Autodesk Fusion 360 part; units mm, degrees
(part 2 of 2)
sketch "Skizze6 (2)" plane through (0, 6, 0) normal (0, -1, 0) x (1, 0, 0) in component "cutouts"
  line L0 (82, 5) -> (172, 5)
  line L1 (172, 5) -> (172, 50)
  line L2 (172, 50) -> (82, 50)
  line L3 (82, 50) -> (82, 5)
  line L4 (87, 10) -> (167, 10)
  line L5 (167, 10) -> (167, 45)
  line L6 (167, 45) -> (87, 45)
  line L7 (87, 45) -> (87, 10)
  line L8 (92.4157, 47.7212) -> (96.4157, 47.7212)
  line L9 (96.4157, 47.7212) -> (96.4157, 6.7721)
  line L10 (96.4157, 6.7721) -> (92.4157, 6.7721)
  line L11 (92.4157, 6.7721) -> (92.4157, 47.7212)
  line L12 (105.7014, 47.7212) -> (105.7014, 6.7721)
  line L13 (101.7014, 6.7721) -> (101.7014, 47.7212)
  line L14 (114.9871, 47.7212) -> (114.9871, 6.7721)
  line L15 (110.9871, 6.7721) -> (110.9871, 47.7212)
  line L16 (124.2728, 47.7212) -> (124.2728, 6.7721)
  line L17 (120.2728, 6.7721) -> (120.2728, 47.7212)
  line L18 (133.5585, 47.7212) -> (133.5585, 6.7721)
  line L19 (129.5585, 6.7721) -> (129.5585, 47.7212)
  line L20 (142.8443, 47.7212) -> (142.8443, 6.7721)
  line L21 (138.8443, 6.7721) -> (138.8443, 47.7212)
  line L22 (152.13, 47.7212) -> (152.13, 6.7721)
  line L23 (148.13, 6.7721) -> (148.13, 47.7212)
  line L24 (161.4157, 47.7212) -> (161.4157, 6.7721)
  line L25 (157.4157, 6.7721) -> (157.4157, 47.7212)
  line L26 (157.4157, 36) -> (105.7014, 36)
  line L27 (105.7014, 40) -> (157.4157, 40)
  line L28 (0, 10) -> (178, 10)
  dimension "d245" = -5
  dimension "d246" = 4
  dimension "d249" = 65
  dimension "d250" = 0
  dimension "d405" = 4
  dimension "d408" = 3.2279
  dimension "d409" = 5
  constraint horizontal L8
  constraint vertical L9
  constraint horizontal L10
  constraint vertical L11
  constraint coincident L25 L26.start
  constraint perpendicular L16 L26
  constraint coincident L25 L27.end
  constraint perpendicular L25 L27
  constraint coincident L12 L26.end
  measures "d246" distance of L8.start L8.end
  measures "d405" distance of L26.end L27.start
  measures "d408" distance of L10 L28
  measures "d409" distance of L6 L27
extrude "Extrusion8'''" cut sketch "Skizze6 (2)" against normal blind 10 contours L4 L6 L7 L11 L28 | L4 L5 L6 L24 L28 | L4 L6 L9 L13 L28 | L4 L22 L25 L26 L28 | L4 L22 L23 L26 L28 | L6 L22 L25 L27 | L4 L12 L15 L26 L28 | L4 L20 L23 L26 L28 | L12 L15 L26 L27 | L6 L12 L15 L27 | L4 L20 L21 L26 L28 | L6 L20 L23 L27 | L4 L14 L17 L26 L28 | L4 L18 L21 L26 L28 | L4 L16 L17 L26 L28 | L6 L14 L17 L27 | L4 L18 L19 L26 L28 | L6 L18 L21 L27 | L4 L16 L19 L26 L28 | L6 L16 L19 L27 bodies 5 in component "computer-case"
sketch "Skizze7" plane through (82, 0, 0) normal (-1, 0, 0) x (0, -1, 0) in component "cutouts"
  line L0 (-19.5, 8) -> (-19.5, 28)
  line L1 (-19.5, 28) -> (-9, 28)
  line L2 (-9, 28) -> (-9, 8)
  line L3 (-9, 8) -> (-19.5, 8)
  line L4 (-169, 5) -> (-6, 5)
  line L5 (-6, 5) -> (-6, 50)
  line L6 (-6, 50) -> (-169, 50)
  line L7 (-169, 50) -> (-169, 5)
  line L8 (-137.7003, 5) -> (-137.7003, 50)
  line L9 (-166, 13) -> (-146, 13)
  line L10 (-146, 13) -> (-146, 33)
  line L11 (-146, 33) -> (-166, 33)
  line L12 (-166, 33) -> (-166, 13)
  dimension "d253" = 20
  dimension "d254" = 20
  dimension "d255" = 8
  dimension "d256" = 3
  constraint horizontal L9
  constraint vertical L10
  constraint horizontal L11
  constraint vertical L12
  measures "d253" distance of L9.start L9.end
  measures "d254" distance of L9.start L11.end
  measures "d255" distance of L4 L9.start
  measures "d256" distance of L7 L12
extrude "Extrusion10''" cut sketch "Skizze7" along normal blind 14 from surface at -10 contours L9 L10 L11 L12 bodies 7 in component "power-supply"
extrude "Extrusion9''" cut sketch "Skizze7" along normal blind 14 from surface at -10 contours L9 L10 L11 L12 bodies 5 in component "computer-case"
sketch "Skizze8" plane through (0, 137.7003, 0) normal (0, 1, 0) x (-1, 0, 0) in component "cutouts"
  line L0 (-81, 5) -> (-6, 5)
  line L1 (-6, 5) -> (-6, 50)
  line L2 (-6, 50) -> (-81, 50)
  line L3 (-81, 50) -> (-81, 5)
  line L4 (-66, 28) -> (-21, 28)
  line L5 (-21, 28) -> (-21, 8)
  line L6 (-21, 8) -> (-66, 8)
  line L7 (-66, 8) -> (-66, 28)
  line L8 (-21, 28) -> (-6, 28) construction
  line L9 (-66, 28) -> (-81, 28) construction
  circle A0 centre (-77.5, 8.5) radius 1
  circle A1 centre (-9.5, 8.5) radius 1
  circle A2 centre (-77.5, 8.5) radius 2.5
  circle A3 centre (-9.5, 8.5) radius 2.5
  dimension "d287" = 45
  dimension "d288" = 20
  dimension "d289" = 3
  dimension "d296" = 5
  dimension "d297" = 5
  constraint horizontal L4
  constraint vertical L5
  constraint horizontal L6
  constraint vertical L7
  constraint coincident L1 L8.end
  constraint perpendicular L1 L8
  constraint coincident L3 L9.end
  constraint perpendicular L3 L9
  constraint equal L8 L9
  constraint concentric A0 A2
  constraint concentric A1 A3
  measures "d287" distance of L4.start L4.end
  measures "d288" distance of L4.start L6.end
  measures "d289" distance of L0 L6
  measures "d296" diameter of A2
  measures "d297" diameter of A3
extrude "Extrusion15" cut sketch "Skizze8" along normal blind 15 from surface at -8 contours L4 L5 L6 L7 bodies 2 in component "light-controller-case"
extrude "Extrusion11'" cut sketch "Skizze8" along normal blind 15 from surface at -8 contours L4 L5 L6 L7 bodies 8 in component "power-supply"
extrude "Extrusion16" cut sketch "Skizze8" against normal blind 2 contours A0 | A1 | A2 | A3 bodies 2 in component "light-controller-case"
sketch "Skizze4 (4)" plane through (0, 0, 113) normal (0, 0, 1) x (-1, 0, 0) in component "fan-holder"
  line L0 (-13.419, -136.793) -> (-138.419, -136.793)
  line L1 (-138.419, -136.793) -> (-138.419, -162.9077)
  line L2 (-138.419, -162.9077) -> (-82, -162.9077)
  line L3 (-82, -162.9077) -> (-82, -137.7003)
  line L4 (-82, -137.7003) -> (-13.419, -137.7003)
  line L5 (-13.419, -137.7003) -> (-13.419, -136.793)
  ellipse E0 centre (-75.919, -81.793) end of major axis (-132.919, -81.793) minor radius 50.9823
  line L6 (-138.419, -26.793) -> (-138.419, -136.793)
  line L7 (-138.419, -136.793) -> (-13.419, -136.793)
  line L8 (-13.419, -136.793) -> (-13.419, -26.793)
  line L9 (-13.419, -26.793) -> (-138.419, -26.793)
  line L10 (-133.419, -31.793) -> (-133.419, -131.793) construction
  line L11 (-133.419, -131.793) -> (-18.419, -131.793) construction
  line L12 (-18.419, -131.793) -> (-18.419, -31.793) construction
  line L13 (-18.419, -31.793) -> (-133.419, -31.793) construction
  circle A0 centre (-133.419, -131.793) radius 1
  circle A1 centre (-18.419, -131.793) radius 1
  circle A2 centre (-18.419, -31.793) radius 1
  circle A3 centre (-133.419, -31.793) radius 1
  ellipse E1 centre (-127.919, -35.2828) end of major axis (-128.919, -35.2828) minor radius 0.8944
  ellipse E2 centre (-127.919, -128.3032) end of major axis (-128.919, -128.3032) minor radius 0.8944
  ellipse E3 centre (-23.919, -35.2828) end of major axis (-24.919, -35.2828) minor radius 0.8944
  ellipse E4 centre (-23.919, -128.3032) end of major axis (-24.919, -128.3032) minor radius 0.8944
  circle A4 centre (-18.419, -131.793) radius 2.5
  circle A5 centre (-133.419, -131.793) radius 2.5
  circle A6 centre (-133.419, -31.793) radius 2.5
  circle A7 centre (-18.419, -31.793) radius 2.5
  dimension "d300" = -5
  dimension "d301" = 2
  dimension "d302" = 2
  dimension "d303" = 2
  dimension "d304" = 2
  dimension "d315" = 5
  dimension "d316" = 5
  dimension "d317" = 5
  dimension "d318" = 5
  constraint coincident L10.end L11.start
  constraint coincident L11.end L12.start
  constraint coincident L12.end L13.start
  constraint coincident L10.start L13.end
  constraint concentric A1 A4
  constraint concentric A0 A5
  constraint concentric A3 A6
  constraint concentric A2 A7
  measures "d301" diameter of A0
  measures "d302" diameter of A1
  measures "d303" diameter of A2
  measures "d304" diameter of A3
  measures "d315" diameter of A4
  measures "d316" diameter of A5
  measures "d317" diameter of A6
  measures "d318" diameter of A7
extrude "Extrusion4'''" cut sketch "Skizze4 (4)" against normal blind 55 contours A0 | A1 | A2 | A3 | A4 | A5 | A6 | A7 bodies 9 in component "fan-holder"
extrude "Extrusion18" cut sketch "Skizze4 (4)" against normal blind 70 contours A0 | A1 | A2 | A3 bodies 4 in component "light-controller-case"
extrude "Extrusion11''" cut sketch "Skizze4 (4)" against normal blind 70 contours A0 | A1 | A2 | A3 bodies 6 in component "computer-case"
extrude "Extrusion5'''" cut sketch "Skizze4 (4)" against normal blind 70 contours A0 | A1 | A2 | A3 bodies 9 in component "fan-holder"
extrude "Extrusion9'''" cut sketch "Skizze2 (3)" against normal blind 20 contours L26 L27 L28 L29 bodies 1 in component "case"
extrude "Extrusion12'" cut sketch "Skizze2 (3)" against normal blind 20 contours L26 L27 L28 L29 bodies 7 in component "power-supply"
sketch "Skizze9" plane through (0, 138.7003, 0) normal (0, -1, 0) x (1, 0, 0) in component "cutouts"
  line L0 (66, 28) -> (66, 8)
  line L1 (66, 8) -> (21, 8)
  line L2 (21, 8) -> (21, 28)
  line L3 (21, 28) -> (66, 28)
  line L4 (47.5027, 53) -> (47.5027, 93.0501)
  spline S0 degree 3 poles (47.5027, 93.0501) (47.5194, 93.0724) (47.5362, 93.0947) (47.553, 93.117) (49.0347, 95.0847) (50.6133, 96.9794) (52.3027, 98.7588) knots -4.432405 -4.432405 -4.432405 -4.432405 -4.42386 -4.42386 -4.42386 -3.669325 -3.669325 -3.669325 -3.669325
  line L5 (44.5027, 88.7668) -> (44.5027, 53)
  line L6 (44.5027, 53) -> (39.7027, 53)
  line L7 (39.7027, 53) -> (39.7027, 80.5615)
  spline S1 degree 3 poles (39.7027, 80.5615) (40.3231, 81.743) (40.9644, 82.9128) (42.5424, 85.6635) (43.4988, 87.232) (44.5027, 88.7668) knots -5.933426 -5.933426 -5.933426 -5.933426 -5.526632 -5.526632 -4.965959 -4.965959 -4.965959 -4.965959
  line L8 (60.1027, 53) -> (55.3027, 53)
  line L9 (55.3027, 53) -> (55.3027, 101.6818)
  spline S2 degree 3 poles (55.3027, 101.6818) (55.3993, 101.7685) (55.4962, 101.8548) (56.7256, 102.9409) (57.9048, 103.8871) (59.4535, 104.9916) (59.7765, 105.2148) (60.1027, 105.4328) knots -3.239152 -3.239152 -3.239152 -3.239152 -3.199117 -3.199117 -2.733019 -2.733019 -2.611699 -2.611699 -2.611699 -2.611699
  line L10 (36.7027, 74.4264) -> (36.7027, 53)
  line L11 (36.7027, 53) -> (31.9027, 53)
  line L12 (31.9027, 53) -> (31.9027, 62.5142)
  spline S3 degree 3 poles (31.9027, 62.5142) (33.2964, 66.4358) (34.8355, 70.2996) (36.5988, 74.198) (36.6507, 74.3123) (36.7027, 74.4264) knots -7.929108 -7.929108 -7.929108 -7.929108 -6.665095 -6.665095 -6.626914 -6.626914 -6.626914 -6.626914
  line L13 (63.1027, 53) -> (63.1027, 107.2351)
  line L14 (76, 108) -> (76, 53)
  line L15 (67.9027, 53) -> (63.1027, 53)
  circle A0 centre (9.5, 109.5) radius 1
  circle A1 centre (9.5, 8.5) radius 1
  circle A2 centre (77.5, 109.5) radius 1
  circle A3 centre (77.5, 8.5) radius 1
  line L16 (6, 5) -> (81, 5)
  line L17 (81, 5) -> (81, 113)
  line L18 (81, 113) -> (6, 113)
  line L19 (6, 113) -> (6, 5)
  line L20 (6, 53) -> (81, 53)
  line L21 (11, 55) -> (21, 55)
  line L22 (21, 55) -> (21, 62)
  line L23 (21, 62) -> (11, 62)
  line L24 (11, 62) -> (11, 55)
  line L25 (64.6301, 108) -> (67.9027, 108)
  line L26 (52.3027, 98.7588) -> (52.3027, 53)
  line L27 (52.3027, 53) -> (47.5027, 53)
  line L28 (60.1027, 105.4328) -> (60.1027, 53)
  spline S4 degree 3 poles (63.1027, 107.2351) (63.6055, 107.5036) (64.1147, 107.759) (64.6301, 108) knots -2.249901 -2.249901 -2.249901 -2.249901 -2.072733 -2.072733 -2.072733 -2.072733
  line L29 (67.9027, 108) -> (67.9027, 53)
  line L30 (76, 53) -> (70.9027, 53)
  line L31 (70.9027, 53) -> (70.9027, 108)
  line L32 (70.9027, 108) -> (76, 108)
  dimension "d333" = 10
  dimension "d334" = 7
  dimension "d335" = 2
  dimension "d336" = 5
  constraint horizontal L21
  constraint vertical L22
  constraint horizontal L23
  constraint vertical L24
  measures "d333" distance of L21.start L21.end
  measures "d334" distance of L21.start L23.end
  measures "d335" distance of L20 L21
  measures "d336" distance of L19 L24
extrude "Extrusion13'" cut sketch "Skizze9" against normal blind 10 contours L21 L22 L23 L24 bodies 8 in component "power-supply"
sketch "Skizze1 (6)" plane through (0, 0, 53) normal (0, 0, 1) x (-1, 0, 0) in component "arduino-mega-case"
  circle A0 centre (-133.419, -31.793) radius 1
  circle A1 centre (-133.419, -131.793) radius 1
  line L0 (-132.5453, -90.7579) -> (-132.5453, -105.3281)
  ellipse E0 centre (-75.919, -98.043) end of major axis (-75.919, -34.3151) minor radius 57 (-132.5453, -90.7579) -> (-132.5453, -105.3281) ccw
  line L1 (-121.2953, -59.4751) -> (-121.2953, -136.6109)
  ellipse E1 centre (-75.919, -98.043) end of major axis (-75.919, -34.3151) minor radius 57 (-128.5453, -122.5244) -> (-121.2953, -136.6109) ccw
  line L2 (-128.5453, -122.5244) -> (-128.5453, -73.5617)
  ellipse E2 centre (-75.919, -98.043) end of major axis (-75.919, -34.3151) minor radius 57 (-121.2953, -59.4751) -> (-128.5453, -73.5617) ccw
  line L3 (-94.7953, -158.175) -> (-94.7953, -37.911)
  ellipse E3 centre (-75.919, -98.043) end of major axis (-75.919, -34.3151) minor radius 57 (-88.0723, -35.7805) -> (-94.7953, -37.911) ccw
  line L4 (-88.0723, -35.7805) -> (-88.0723, -160.3055)
  ellipse E4 centre (-75.919, -98.043) end of major axis (-75.919, -34.3151) minor radius 57 (-94.7953, -158.175) -> (-88.0723, -160.3055) ccw
  line L5 (-110.0453, -46.999) -> (-110.0453, -149.087)
  ellipse E5 centre (-75.919, -98.043) end of major axis (-75.919, -34.3151) minor radius 57 (-117.2953, -141.8751) -> (-110.0453, -149.087) ccw
  line L6 (-117.2953, -141.8751) -> (-117.2953, -54.211)
  ellipse E6 centre (-75.919, -98.043) end of major axis (-75.919, -34.3151) minor radius 57 (-110.0453, -46.999) -> (-117.2953, -54.211) ccw
  line L7 (-98.7953, -39.6727) -> (-98.7953, -156.4133)
  ellipse E7 centre (-75.919, -98.043) end of major axis (-75.919, -34.3151) minor radius 57 (-106.0453, -152.1425) -> (-98.7953, -156.4133) ccw
  line L8 (-106.0453, -152.1425) -> (-106.0453, -43.9435)
  ellipse E8 centre (-75.919, -98.043) end of major axis (-75.919, -34.3151) minor radius 57 (-98.7953, -39.6727) -> (-106.0453, -43.9435) ccw
  ellipse E9 centre (-127.919, -39.9052) end of major axis (-127.919, -38.7872) minor radius 1 (-127.1786, -39.1537) -> (-128.6593, -39.1537) ccw
  line L9 (-127.1786, -39.1537) -> (-128.6593, -39.1537)
  circle A2 centre (-168.5, -165.5) radius 1
  circle A3 centre (-168.5, -9.5) radius 1
  circle A4 centre (-85.5, -9.5) radius 1
  circle A5 centre (-85.5, -165.5) radius 1
  line L10 (-82, -6) -> (-172, -6)
  line L11 (-172, -6) -> (-172, -169)
  line L12 (-172, -169) -> (-82, -169)
  line L13 (-82, -169) -> (-82, -6)
  line L14 (-138.419, -26.793) -> (-138.419, -136.793)
  line L15 (-171, -161.774) -> (-143.419, -161.774)
  line L16 (-143.419, -161.774) -> (-143.419, -26.774)
  line L17 (-143.419, -26.774) -> (-171, -26.774)
  line L18 (-171, -26.774) -> (-171, -161.774)
  line L19 (-168, -158.774) -> (-146.419, -158.774)
  line L20 (-146.419, -158.774) -> (-146.419, -29.774)
  line L21 (-146.419, -29.774) -> (-168, -29.774)
  line L22 (-168, -29.774) -> (-168, -158.774)
  line L23 (-146.419, -29.774) -> (-146.419, -26.774)
  line L24 (-146.419, -158.774) -> (-146.419, -161.774)
  line L25 (-152.0037, -35.3587) -> (-162.4153, -35.3587) construction
  line L26 (-162.4153, -35.3587) -> (-162.4153, -153.1893) construction
  line L27 (-162.4153, -153.1893) -> (-152.0037, -153.1893) construction
  line L28 (-152.0037, -153.1893) -> (-152.0037, -35.3587) construction
  circle A6 centre (-162.4153, -153.1893) radius 1
  circle A7 centre (-152.0037, -153.1893) radius 1
  circle A8 centre (-162.4153, -35.3587) radius 1
  circle A9 centre (-152.0037, -35.3587) radius 1
  circle A10 centre (-162.4153, -35.3587) radius 2.5
  circle A11 centre (-152.0037, -35.3587) radius 2.5
  circle A12 centre (-162.4153, -153.1893) radius 2.5
  circle A13 centre (-152.0037, -153.1893) radius 2.5
  dimension "d339" = 1
  dimension "d340" = 5
  dimension "d341" = 135
  dimension "d342" = 20.774
  dimension "d343" = -3
  dimension "d362" = -8.5847
  dimension "d363" = 2
  dimension "d364" = 2
  dimension "d365" = 2
  dimension "d366" = 2
  dimension "d367" = 5
  dimension "d368" = 5
  dimension "d369" = 5
  dimension "d370" = 5
  constraint horizontal L15
  constraint vertical L16
  constraint horizontal L17
  constraint vertical L18
  constraint coincident L17 L23.end
  constraint perpendicular L17 L23
  constraint coincident L15 L24.end
  constraint perpendicular L15 L24
  constraint coincident L26.end L27.start
  constraint coincident L27.end L28.start
  constraint coincident L25.end L26.start
  constraint coincident L25.start L28.end
  constraint concentric A8 A10
  constraint concentric A9 A11
  constraint concentric A6 A12
  constraint concentric A7 A13
  measures "d339" distance of L11 L18
  measures "d340" distance of L14 L16
  measures "d341" distance of L15.start L17.end
  measures "d342" distance of L10 L17.end
  measures "d363" diameter of A6
  measures "d364" diameter of A7
  measures "d365" diameter of A8
  measures "d366" diameter of A9
  measures "d367" diameter of A10
  measures "d368" diameter of A11
  measures "d369" diameter of A12
  measures "d370" diameter of A13
extrude "Extrusion1''''" add sketch "Skizze1 (6)" along normal blind 60 separate body contours L15 L17 L18 L19 L21 L22 L23 L24 makes body 10 in component "arduino-mega-case"
extrude "Extrusion2''''" add sketch "Skizze1 (6)" along normal blind 3 contours L19 L20 L21 L22 | A6 | A7 | A8 | A9 | A10 | A11 | A12 | A13 bodies 10 in component "arduino-mega-case"
extrude "Extrusion3''''" add sketch "Skizze1 (6)" along normal blind 3 from surface at 60 contours L15 L17 L18 L19 L21 L22 L23 L24 | L19 L20 L21 L22 | A6 | A7 | A8 | A9 | A10 | A11 | A12 | A13 bodies 10 in component "arduino-mega-case"
extrude "Extrusion4''''" add sketch "Skizze1 (6)" along normal blind 63 separate body contours L15 L16 L17 L20 L23 L24 makes body 11 in component "arduino-mega-case"
chamfer "Fase1'''''" distance 6 angle 45 4 edges at (157.2095, 158.774, 56) (157.2095, 158.774, 113) (157.2095, 29.774, 56) (157.2095, 29.774, 113) on bodies 10 in component "arduino-mega-case"
sketch "Skizze3 (4)" plane through (146.419, 0, 0) normal (-1, 0, 0) x (0, -1, 0) in component "arduino-mega-case"
  line L0 (-29.774, 62) -> (-35.774, 56)
  line L1 (-35.774, 56) -> (-152.774, 56)
  line L2 (-152.774, 56) -> (-158.774, 62)
  line L3 (-158.774, 62) -> (-158.774, 107)
  line L4 (-158.774, 107) -> (-152.774, 113)
  line L5 (-152.774, 113) -> (-35.774, 113)
  line L6 (-35.774, 113) -> (-29.774, 107)
  line L7 (-29.774, 107) -> (-29.774, 62)
  line L8 (-26.774, 53) -> (-26.774, 116)
  line L9 (-26.774, 116) -> (-161.774, 116)
  line L10 (-161.774, 116) -> (-161.774, 53)
  line L11 (-161.774, 53) -> (-26.774, 53)
  line L12 (-158.274, 56.5) -> (-30.274, 56.5) construction
  line L13 (-30.274, 56.5) -> (-30.274, 112.5) construction
  line L14 (-30.274, 112.5) -> (-158.274, 112.5) construction
  line L15 (-158.274, 112.5) -> (-158.274, 56.5) construction
  circle A0 centre (-30.274, 112.5) radius 1
  circle A1 centre (-30.274, 56.5) radius 1
  circle A2 centre (-158.274, 56.5) radius 1
  circle A3 centre (-158.274, 112.5) radius 1
  dimension "d354" = -3.5
  dimension "d355" = 2
  dimension "d356" = 2
  dimension "d357" = 2
  dimension "d358" = 2
  constraint coincident L13.end L14.start
  constraint coincident L12.end L13.start
  constraint coincident L12.start L15.end
  constraint coincident L14.end L15.start
  measures "d355" diameter of A0
  measures "d356" diameter of A1
  measures "d357" diameter of A2
  measures "d358" diameter of A3
extrude "Extrusion5''''" cut sketch "Skizze3 (4)" along normal blind 10 from surface at -7 contours A0 | A1 | A2 | A3 bodies 10 11 in component "arduino-mega-case"
extrude "Extrusion6''''" cut sketch "Skizze1 (6)" along normal blind 15 contours A6 | A7 | A8 | A9 bodies 10 in component "arduino-mega-case"
extrude "Extrusion7''''" cut sketch "Skizze1 (6)" along normal blind 11 from surface at 3 contours A10 | A11 | A12 | A13 bodies 10 in component "arduino-mega-case"
sketch "Skizze10" plane through (0, 26.774, 0) normal (0, -1, 0) x (1, 0, 0) in component "cutouts"
  line L0 (146.419, 53) -> (171, 53)
  line L1 (171, 53) -> (171, 116)
  line L2 (171, 116) -> (146.419, 116)
  line L3 (146.419, 116) -> (146.419, 53)
  line L4 (151.419, 111) -> (151.419, 58)
  line L5 (151.419, 58) -> (166, 58)
  line L6 (166, 58) -> (166, 111)
  line L7 (166, 111) -> (151.419, 111)
  dimension "d376" = -5
extrude "Extrusion8''''" cut sketch "Skizze10" against normal blind 10 contours L4 L5 L6 L7 bodies 10 in component "arduino-mega-case"
sketch "Skizze11" plane through (0, 0, 53) normal (0, 0, 1) x (-1, 0, 0) in component "cutouts"
  circle A0 centre (-133.419, -31.793) radius 1
  circle A1 centre (-133.419, -131.793) radius 1
  line L0 (-132.5453, -90.7579) -> (-132.5453, -105.3281)
  ellipse E0 centre (-75.919, -98.043) end of major axis (-75.919, -34.3151) minor radius 57 (-132.5453, -90.7579) -> (-132.5453, -105.3281) ccw
  line L1 (-121.2953, -59.4751) -> (-121.2953, -136.6109)
  ellipse E1 centre (-75.919, -98.043) end of major axis (-75.919, -34.3151) minor radius 57 (-128.5453, -122.5244) -> (-121.2953, -136.6109) ccw
  line L2 (-128.5453, -122.5244) -> (-128.5453, -73.5617)
  ellipse E2 centre (-75.919, -98.043) end of major axis (-75.919, -34.3151) minor radius 57 (-121.2953, -59.4751) -> (-128.5453, -73.5617) ccw
  line L3 (-94.7953, -158.175) -> (-94.7953, -37.911)
  ellipse E3 centre (-75.919, -98.043) end of major axis (-75.919, -34.3151) minor radius 57 (-88.0723, -35.7805) -> (-94.7953, -37.911) ccw
  line L4 (-88.0723, -35.7805) -> (-88.0723, -160.3055)
  ellipse E4 centre (-75.919, -98.043) end of major axis (-75.919, -34.3151) minor radius 57 (-94.7953, -158.175) -> (-88.0723, -160.3055) ccw
  line L5 (-110.0453, -46.999) -> (-110.0453, -149.087)
  ellipse E5 centre (-75.919, -98.043) end of major axis (-75.919, -34.3151) minor radius 57 (-117.2953, -141.8751) -> (-110.0453, -149.087) ccw
  line L6 (-117.2953, -141.8751) -> (-117.2953, -54.211)
  ellipse E6 centre (-75.919, -98.043) end of major axis (-75.919, -34.3151) minor radius 57 (-110.0453, -46.999) -> (-117.2953, -54.211) ccw
  line L7 (-98.7953, -39.6727) -> (-98.7953, -156.4133)
  ellipse E7 centre (-75.919, -98.043) end of major axis (-75.919, -34.3151) minor radius 57 (-106.0453, -152.1425) -> (-98.7953, -156.4133) ccw
  line L8 (-106.0453, -152.1425) -> (-106.0453, -43.9435)
  ellipse E8 centre (-75.919, -98.043) end of major axis (-75.919, -34.3151) minor radius 57 (-98.7953, -39.6727) -> (-106.0453, -43.9435) ccw
  ellipse E9 centre (-127.919, -39.9052) end of major axis (-127.919, -38.7872) minor radius 1 (-127.1786, -39.1537) -> (-128.6593, -39.1537) ccw
  line L9 (-127.1786, -39.1537) -> (-128.6593, -39.1537)
  circle A2 centre (-168.5, -165.5) radius 1
  circle A3 centre (-168.5, -9.5) radius 1
  circle A4 centre (-85.5, -9.5) radius 1
  circle A5 centre (-85.5, -165.5) radius 1
  line L10 (-82, -6) -> (-172, -6)
  line L11 (-172, -6) -> (-172, -169)
  line L12 (-172, -169) -> (-82, -169)
  line L13 (-82, -169) -> (-82, -6)
  line L14 (-166, -26.774) -> (-151.419, -26.774)
  line L15 (-151.419, -26.774) -> (-151.419, -12.193)
  line L16 (-151.419, -12.193) -> (-166, -12.193)
  line L17 (-166, -12.193) -> (-166, -26.774)
  constraint coincident L14.end L15.start
  constraint perpendicular L14 L15
  constraint perpendicular L15 L16
  constraint coincident L14.start L17.end
  constraint equal L14 L15
extrude "Extrusion12''" cut sketch "Skizze11" against normal blind 10 contours L14 L15 L16 L17 bodies 6 in component "computer-case"
sketch "Skizze4 (5)" plane through (168, 0, 0) normal (-1, 0, 0) x (0, -1, 0) in component "arduino-mega-case"
  line L0 (-29.774, 107) -> (-35.774, 113)
  line L1 (-35.774, 113) -> (-152.774, 113)
  line L2 (-152.774, 113) -> (-158.774, 107)
  line L3 (-158.774, 107) -> (-158.774, 62)
  line L4 (-158.774, 62) -> (-152.774, 56)
  line L5 (-152.774, 56) -> (-35.774, 56)
  line L6 (-35.774, 56) -> (-29.774, 62)
  line L7 (-29.774, 62) -> (-29.774, 107)
  circle A0 centre (-158.274, 112.5) radius 1
  circle A1 centre (-158.274, 56.5) radius 1
  circle A2 centre (-30.274, 112.5) radius 1
  circle A3 centre (-30.274, 56.5) radius 1
  line L8 (-29.774, 62) -> (-35.774, 56)
  line L9 (-35.774, 56) -> (-152.774, 56)
  line L10 (-152.774, 56) -> (-158.774, 62)
  line L11 (-158.774, 62) -> (-158.774, 107)
  line L12 (-158.774, 107) -> (-152.774, 113)
  line L13 (-152.774, 113) -> (-35.774, 113)
  line L14 (-35.774, 113) -> (-29.774, 107)
  line L15 (-29.774, 107) -> (-29.774, 62)
  line L16 (-26.774, 53) -> (-26.774, 116)
  line L17 (-26.774, 116) -> (-161.774, 116)
  line L18 (-161.774, 116) -> (-161.774, 53)
  line L19 (-161.774, 53) -> (-26.774, 53)
  line L20 (-50.6836, 57.87) -> (-151.9836, 57.87) construction
  line L21 (-151.9836, 57.87) -> (-151.9836, 111.13) construction
  line L22 (-151.9836, 111.13) -> (-50.6836, 111.13) construction
  line L23 (-50.6836, 111.13) -> (-50.6836, 57.87) construction
  line L24 (-50.6836, 57.87) -> (-151.9836, 111.13) construction
  line L25 (-151.9836, 57.87) -> (-50.6836, 111.13) construction
  line L26 (-161.774, 84.5) -> (-26.774, 84.5) construction
  line L27 (-151.9836, 60.11) -> (-50.6836, 60.11) construction
  line L28 (-151.9836, 108.75) -> (-50.6836, 108.75) construction
  circle A4 centre (-64.9936, 108.75) radius 1
  circle A5 centre (-65.6836, 60.11) radius 1
  circle A6 centre (-140.7036, 60.11) radius 1
  circle A7 centre (-147.3336, 108.75) radius 1
  point P0 (-101.3336, 84.5)
  dimension "d381" = 101.3
  dimension "d382" = 53.26
  dimension "d383" = 2.24
  dimension "d384" = 2.38
  dimension "d385" = 2
  dimension "d386" = 2
  dimension "d387" = 2
  dimension "d388" = 2
  dimension "d389" = 14.31
  dimension "d390" = 15
  dimension "d391" = 4.65
  dimension "d392" = 11.28
  constraint horizontal L20
  constraint perpendicular L20 L21
  constraint parallel L20 L22
  constraint parallel L21 L23
  constraint coincident L24 P0
  constraint coincident L25 P0
  constraint midpoint L18 L26.start
  constraint midpoint L16 L26.end
  constraint coincident L21 L27.start
  constraint coincident L23 L27.end
  constraint perpendicular L23 L27
  constraint coincident L21 L28.start
  constraint coincident L23 L28.end
  constraint perpendicular L23 L28
  constraint coincident L28 A4.centre
  constraint coincident L27 A5.centre
  constraint coincident L27 A6.centre
  constraint coincident L28 A7.centre
  measures "d381" distance of L21.end L22.end
  measures "d382" distance of L20.end L21.end
  measures "d383" distance of L20 L27
  measures "d384" distance of L22 L28
  measures "d385" diameter of A4
  measures "d386" diameter of A5
  measures "d387" diameter of A6
  measures "d388" diameter of A7
  measures "d389" distance of L28.end A4.centre
  measures "d390" distance of L27.end A5.centre
  measures "d391" distance of L28.start A7.centre
  measures "d392" distance of L27.start A6.centre
extrude "Extrusion9''''" cut sketch "Skizze4 (5)" against normal blind 15 contours A4 | A5 | A6 | A7 bodies 10 in component "arduino-mega-case"
sketch "Skizze5 (3)" plane through (0, 169, 0) normal (0, 1, 0) x (-1, 0, 0) in component "computer-case"
  line L0 (-172, 5) -> (-82, 5)
  line L1 (-82, 5) -> (-82, 50)
  line L2 (-82, 50) -> (-172, 50)
  line L3 (-172, 50) -> (-172, 5)
  line L4 (-162, 36) -> (-92, 36)
  line L5 (-92, 36) -> (-92, 8)
  line L6 (-92, 8) -> (-162, 8)
  line L7 (-162, 8) -> (-162, 36)
  dimension "d395" = 3
  dimension "d396" = 14
  dimension "d397" = 10
  dimension "d398" = 10
  constraint horizontal L4
  constraint vertical L5
  constraint horizontal L6
  constraint vertical L7
  measures "d395" distance of L0 L6
  measures "d396" distance of L2 L4
  measures "d397" distance of L1 L5
  measures "d398" distance of L3 L7
extrude "Extrusion10'''" cut sketch "Skizze5 (3)" along normal blind 20 from surface at -5 contours L4 L5 L6 L7 bodies 1 in component "case"
extrude "Extrusion13''" cut sketch "Skizze5 (3)" along normal blind 20 from surface at -5 contours L4 L5 L6 L7 bodies 5 in component "computer-case"
extrude "Extrusion14'" cut 1 faces at (36, 140.7003, 8) along direction (0, 0, -1) blind 6 on bodies 8 bodies 8 in component "power-supply"
component "case" placed x (1, 0, 0) y (0, 1, 0) z (0, 0, 1) at (0, 0, 0)
component "light-controller-case" placed x (1, 0, 0) y (0, 1, 0) z (0, 0, 1) at (0, 0, 0)
component "computer-case" placed x (1, 0, 0) y (0, 1, 0) z (0, 0, 1) at (0, 0, 0)
component "power-supply" placed x (1, 0, 0) y (0, 1, 0) z (0, 0, 1) at (0, 0, 0)
component "fan-holder" placed x (1, 0, 0) y (0, 1, 0) z (0, 0, 1) at (0, 0, 0)
component "cutouts" placed x (1, 0, 0) y (0, 1, 0) z (0, 0, 1) at (0, 0, 0)
component "arduino-mega-case" placed x (1, 0, 0) y (0, 1, 0) z (0, 0, 1) at (0, 0, 0)
equation "d8 = 122 mm - 6 mm"
equation "d11 = 112.00 mm - 6 mm"
equation "d50 = 25.00 mm + 3 mm + 17 mm"
equation "screw_hole_size = 2 mm"
equation "d81 = screw_hole_size"
equation "d82 = screw_hole_size"
equation "d83 = screw_hole_size"
equation "d84 = screw_hole_size"
equation "d133 = screw_hole_size"
equation "d134 = screw_hole_size"
equation "d135 = screw_hole_size"
equation "d136 = screw_hole_size"
equation "d164 = screw_hole_size"
equation "d165 = screw_hole_size"
equation "d166 = screw_hole_size"
equation "d167 = screw_hole_size"
equation "d172 = screw_hole_size"
equation "d173 = screw_hole_size"
equation "d174 = screw_hole_size"
equation "d175 = screw_hole_size"
equation "d178 = 105.00 mm + 3 mm"
equation "d305 = screw_hole_size"
equation "d306 = screw_hole_size"
equation "d307 = screw_hole_size"
equation "d308 = screw_hole_size"
equation "d344 = 3 mm + 57 mm"
equation "d351 = 6 mm + 57 mm"
equation "d385 = screw_hole_size"
equation "d386 = screw_hole_size"
equation "d387 = screw_hole_size"
equation "d388 = screw_hole_size"
named bodies: "box", "plate", "top-plate", "top"
